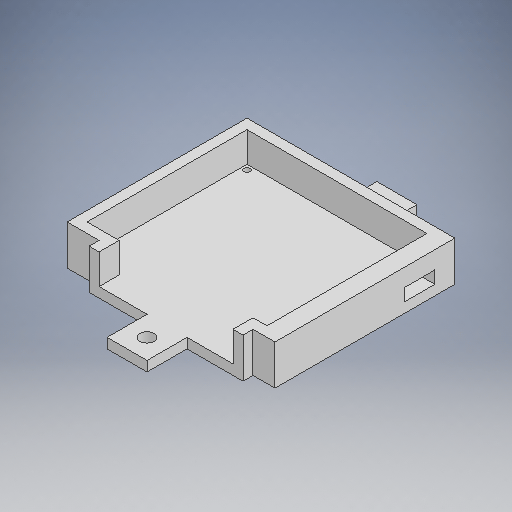
# Autodesk Inventor part: imu_case_new
Saved by Autodesk Inventor 2025.2 (Build 292293000, 293)
## iProperties
Created: 2025-01-20
Part Number: imu_case_new
Material: 일반
Document SubType Name: Sheet Metal
Designer: 1dnlc
Density: 1 g/cm^3
Sheet Metal Rule: 기본값_mm
Appearance: 기본값
Author: 1dnlc
Autodesk Inventor part; units mm, degrees
ref_plane "YZ Plane" through (0, 0, 0) normal (1, 0, 0) x (0, 1, 0)
ref_plane "XZ Plane" through (0, 0, 0) normal (0, 1, 0) x (-1, 0, 0)
ref_plane "XY Plane" through (0, 0, 0) normal (0, 0, 1) x (1, 0, 0)
sketch "스케치1" plane through (0, 0, 0) normal (0, 1, 0) x (-1, 0, 0)
  line L0 (0, 0) -> (104, 0)
  line L1 (104, 0) -> (104, -90)
  line L2 (104, -90) -> (0, -90)
  line L3 (0, -90) -> (0, 0)
  line L4 (59, -90) -> (39, -90)
  line L5 (39, -90) -> (39, -110)
  line L6 (39, -110) -> (59, -110)
  line L7 (59, -110) -> (59, -90)
  line L8 (88, 0) -> (11, 0)
  line L9 (11, 0) -> (11, 5)
  line L10 (11, 5) -> (88, 5)
  line L11 (88, 5) -> (88, 0)
  line L12 (39, 5) -> (59, 5)
  line L13 (59, 5) -> (59, 25)
  line L14 (59, 25) -> (39, 25)
  line L15 (39, 25) -> (39, 5)
  point P0 (49, -110)
  point P1 (11, 2.5)
  point P2 (88, 2.5)
  dimension "d0" = 90
  dimension "d1" = 104
  dimension "d2" = 39
  dimension "d3" = 59
  dimension "d4" = 20
  dimension "d5" = 5
  dimension "d6" = 11
  dimension "d7" = 16
  dimension "d8" = 39
  dimension "d9" = 59
  dimension "d10" = 20
  constraints: 32 end point, 8 parallel, 4 horizontal, 4 perpendicular, 3 midpoint, 3 point on line
  measures "d0" distance between parallel lines of L2 L0
  measures "d1" distance between parallel lines of L3 L1
  measures "d2" distance between parallel lines of L3 L5
  measures "d3" distance between parallel lines of L3 L7
  measures "d4" distance from line of point (49, -110) L2
  measures "d5" distance between parallel lines of L0 L10
  measures "d6" distance from line of L3 point (11, 2.5)
  measures "d7" distance from line of L1 point (88, 2.5)
  measures "d8" distance between parallel lines of L3 L15
  measures "d9" distance between parallel lines of L3 L13
  measures "d10" distance between parallel lines of L10 L14
extrude "돌출1" add sketch "스케치1" along normal blind 5
sketch "스케치2" plane through (0, 5, 0) normal (0, 1, 0) x (1, 0, 0)
  line L0 (-88, -5) -> (-59, -5) projected
  line L1 (-88, -5) -> (-83, -5)
  line L2 (-83, -5) -> (-83, 5)
  line L3 (-83, 5) -> (-88, 5)
  line L4 (-88, 5) -> (-88, -5)
  line L5 (-104, 90) -> (-104, 0) projected
  line L6 (-104, 0) -> (-83, 0)
  line L7 (-83, 0) -> (-83, 5)
  line L8 (-83, 5) -> (-104, 5)
  line L9 (-104, 5) -> (-104, 0)
  line L10 (-104, 0) -> (-88, 0) projected
  line L11 (-59, 90) -> (-104, 90) projected
  line L12 (-104, 0) -> (-99, 0)
  line L13 (-99, 0) -> (-99, 90)
  line L14 (-99, 90) -> (-104, 90)
  line L15 (-104, 90) -> (-104, 0)
  line L16 (-104, 90) -> (0, 90)
  line L17 (0, 90) -> (0, 85)
  line L18 (0, 85) -> (-104, 85)
  line L19 (-104, 85) -> (-104, 90)
  line L20 (0, 90) -> (-5.4966, 90)
  line L21 (-39, -5) -> (-11, -5) projected
  line L22 (-11, -5) -> (-16.7717, -5)
  line L23 (-11, -5) -> (-16, -5)
  line L24 (-16, -5) -> (-16, 6.6946)
  line L25 (-11, 6.6946) -> (-11, -5)
  line L26 (-11, 0) -> (0, 0) projected
  line L27 (0, 0) -> (-5, 0)
  line L28 (-5, 0) -> (-5, 90)
  line L29 (-5, 90) -> (0, 90)
  line L30 (0, 90) -> (0, 0)
  line L31 (0, 0) -> (-16, 0)
  line L32 (-16, 0) -> (-16, 5)
  line L33 (-16, 5) -> (0, 5)
  line L34 (0, 5) -> (0, 0)
  point P0 (-88, 0)
  point P1 (-99, 5)
  point P2 (-99, 85)
  point P3 (-5, 85)
  point P4 (-5, 5)
  dimension "d13" = 5
  dimension "d14" = 5
  dimension "d15" = 5
  dimension "d16" = 5
  dimension "d17" = 5
  dimension "d18" = 5
  dimension "d19" = 5
  constraints: 58 end point, 13 parallel, 9 horizontal, 7 perpendicular, 3 point on line
  measures "d13" distance between parallel lines of L13 L5
  measures "d14" distance between parallel lines of L11 L18
  measures "d15" distance between parallel lines of L10 L8
  measures "d16" distance between parallel lines of L4 L2
  measures "d17" distance of L24.end L25.start
  measures "d18" distance of L28.end L29.end
  measures "d19" distance of L31.end L32.end
extrude "돌출2" add sketch "스케치2" along normal blind 15
sketch "스케치4" plane through (0, 5, 0) normal (0, 1, 0) x (1, 0, 0)
  line L0 (-59, 90) -> (-104, 90) projected
  line L1 (-39, 110) -> (-59, 110) projected
  line L2 (-59, 90) -> (-39, 110)
  line L3 (-59, 110) -> (-59, 90) projected
  line L4 (-59, -25) -> (-39, -25) projected
  line L5 (-39, -25) -> (-39, -5) projected
  line L6 (-59, -25) -> (-39, -5)
  line L7 (-83, -5) -> (-59, -5) projected
  line L8 (-39, -25) -> (-59, -5)
  circle A0 centre (-49, -15) radius 3.5
  circle A1 centre (-49, 100) radius 3.5
  line L9 (-39, 90) -> (-39, 110) projected
  line L10 (-59, 110) -> (-39, 90)
  point P0 (0, 0)
  dimension "d23" = 7
  dimension "d24" = 7
  constraints: 8 end point, 2 centre point, 2 midpoint
  measures "d23" diameter of A0
  measures "d24" diameter of A1
extrude "돌출3" cut sketch "스케치4" against normal blind 15 contours A1 L10 L2 | L2 L10 A1 | L10 L2 A1 | L10 A1 L2 | A0 L8 L6 | L6 L8 A0 | L8 L6 A0 | L8 A0 L6
sketch "스케치5" plane through (0, 5, 0) normal (0, 1, 0) x (1, 0, 0)
  line L0 (-5, 5) -> (-5, 85) projected
  line L1 (-5, 85) -> (-99, 85) projected
  line L2 (-5, 5) -> (-8, 5)
  line L3 (-8, 5) -> (-8, 85)
  line L4 (-8, 85) -> (-5, 85)
  line L5 (-5, 85) -> (-5, 5)
  line L6 (0, 0) -> (0, 90) projected
  dimension "d27" = 8
  constraints: 8 end point, 2 parallel, 1 horizontal, 1 perpendicular, 1 point on line
  measures "d27" distance between parallel lines of L6 L3
extrude "돌출4" add sketch "스케치5" along normal blind 15
sketch "스케치6" plane through (0, 5, 0) normal (0, 1, 0) x (1, 0, 0)
  circle A0 centre (-96.5, 7.5) radius 1.5
  circle A1 centre (-96.5, 82.5) radius 1.5
  circle A2 centre (-10.5, 82.5) radius 1.5
  circle A3 centre (-10.5, 7.5) radius 1.5
  line L0 (-83, 5) -> (-99, 5) projected
  line L1 (-99, 5) -> (-99, 85) projected
  line L2 (-99, 85) -> (-8, 85) projected
  line L3 (-8, 85) -> (-8, 5) projected
  line L4 (-8, 5) -> (-16, 5) projected
  point P0 (0, 0)
  dimension "d30" = 3
  dimension "d31" = 3
  dimension "d32" = 3
  dimension "d33" = 3
  dimension "d34" = 2.5
  dimension "d35" = 2.5
  dimension "d36" = 2.5
  dimension "d37" = 2.5
  dimension "d38" = 2.5
  dimension "d39" = 2.5
  dimension "d40" = 2.5
  dimension "d41" = 2.5
  constraints: 4 centre point
  measures "d30" diameter of A0
  measures "d31" diameter of A1
  measures "d32" diameter of A2
  measures "d33" diameter of A3
  measures "d34" distance from line of L0 A0.centre
  measures "d35" distance from line of A0.centre L1
  measures "d36" distance from line of A1.centre L1
  measures "d37" distance from line of L2 A1.centre
  measures "d38" distance from line of L2 A2.centre
  measures "d39" distance from line of L3 A2.centre
  measures "d40" distance from line of L4 A3.centre
  measures "d41" distance from line of L3 A3.centre
extrude "돌출5" cut sketch "스케치6" against normal blind 30
sketch "스케치7" plane through (0, 0, 0) normal (1, 0, 0) x (0, 0, -1)
  line L0 (65, 11.2) -> (80, 11.2)
  line L1 (80, 11.2) -> (80, 5)
  line L2 (80, 5) -> (65, 5)
  line L3 (65, 5) -> (65, 11.2)
  line L4 (0, 0) -> (90, 0) projected
  line L5 (90, 0) -> (90, 20) projected
  point P0 (80, 8.1)
  dimension "d44" = 5
  dimension "d45" = 10
  dimension "d46" = 6.2
  dimension "d47" = 15
  constraints: 8 end point, 2 parallel, 1 horizontal, 1 midpoint, 1 perpendicular
  measures "d44" distance between parallel lines of L4 L2
  measures "d45" distance from line of L5 point (80, 8.1)
  measures "d46" distance between parallel lines of L2 L0
  measures "d47" distance between parallel lines of L1 L3
extrude "돌출6" cut sketch "스케치7" against normal blind 30
sketch "스케치9" plane through (0, 5, 0) normal (0, 1, 0) x (1, 0, 0)
  circle A0 centre (-10.5, 7.5) radius 1.5 projected
  circle A1 centre (-10.5, 7.5) radius 1.5
  circle A2 centre (-10.5, 82.5) radius 1.5 projected
  circle A3 centre (-10.5, 82.5) radius 1.5
  point P0 (0, 0)
  constraints: 2 centre point, 2 coincident
extrude "돌출7" add sketch "스케치9" against normal blind 5
sketch "스케치10" plane through (0, 5, 0) normal (0, 1, 0) x (1, 0, 0)
  line L0 (-8, 85) -> (-8, 5) projected
  line L1 (-8, 85) -> (-99, 85) projected
  line L2 (-8, 5) -> (-9, 5)
  line L3 (-9, 5) -> (-9, 85)
  line L4 (-9, 85) -> (-8, 85)
  line L5 (-8, 85) -> (-8, 5)
  point P0 (0, 0)
  dimension "d52" = 1
  constraints: 8 end point, 2 parallel, 1 horizontal, 1 perpendicular, 1 point on line
  measures "d52" distance of L3.end L4.end
extrude "돌출8" add sketch "스케치10" along normal blind 15
sketch "스케치11" plane through (-8, 5, -65) normal (1, 0, 0) x (0, 0, -1)
  line L0 (0, 0) -> (0, 6.2) projected
  line L1 (15, 6.2) -> (15, 0) projected
  line L2 (0, 6.2) -> (15, 6.2)
  line L3 (15, 6.2) -> (15, 0)
  line L4 (15, 0) -> (0, 0)
  line L5 (0, 0) -> (0, 6.2)
  point P0 (-65, -5)
  constraints: 8 end point, 2 parallel, 1 horizontal, 1 perpendicular
extrude "돌출9" cut sketch "스케치11" against normal blind 15
sketch "스케치12" plane through (0, 5, 0) normal (0, 1, 0) x (1, 0, 0)
  circle A0 centre (-11.5, 7.5) radius 1.5
  circle A1 centre (-11.5, 82.5) radius 1.5
  line L0 (-9, 85) -> (-9, 5) projected
  line L1 (-9, 5) -> (-16, 5) projected
  line L2 (-99, 85) -> (-9, 85) projected
  point P0 (0, 0)
  dimension "d57" = 3
  dimension "d58" = 3
  dimension "d59" = 2.5
  dimension "d60" = 2.5
  dimension "d61" = 2.5
  dimension "d62" = 2.5
  constraints: 2 centre point
  measures "d57" diameter of A0
  measures "d58" diameter of A1
  measures "d59" distance from line of L0 A0.centre
  measures "d60" distance from line of L1 A0.centre
  measures "d61" distance from line of L2 A1.centre
  measures "d62" distance from line of L0 A1.centre
extrude "돌출10" cut sketch "스케치12" against normal blind 15
equation "\"TransitionRadius\" = BendRadius"
equation "\"BendRadius\" = 0.5"
